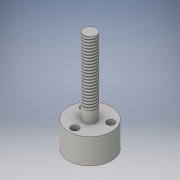
# Autodesk Inventor part: Motor top
Saved by Autodesk Inventor 2016 (Build 200138000, 138)
## iProperties
Created: 2015-05-11
Part Number: Motor top
Material: Generic
Document SubType Name: Modeling
Designer: Admin
Density: 1 g/cm^3
Appearance: Default
Author: Admin
Autodesk Inventor part; units mm, degrees
ref_plane "YZ Plane" through (0, 0, 0) normal (1, 0, 0) x (0, 1, 0)
ref_plane "XZ Plane" through (0, 0, 0) normal (0, 1, 0) x (-1, 0, 0)
ref_plane "XY Plane" through (0, 0, 0) normal (0, 0, 1) x (1, 0, 0)
sketch "Sketch1" plane through (0, 0, 0) normal (0, 1, 0) x (-1, 0, 0)
  circle A0 centre (0, 0) radius 8.5
  circle A1 centre (5.1962, -3) radius 1.5
  circle A2 centre (5.1962, -3) radius 1.5
  circle A3 centre (-5.1962, -3) radius 1.5
  circle A4 centre (-5.1962, -3) radius 1.5
  circle A5 centre (0, 6) radius 1.5
  circle A6 centre (0, 6) radius 1.5
  point P0 (0, 0)
  constraints: 7 centre point, 4 coincident
extrude "Extrusion1" add sketch "Sketch1" along normal blind 10
sketch "Sketch2" plane through (0, 10, 0) normal (0, 1, 0) x (1, 0, 0)
  circle A0 centre (0, 0) radius 2.5
  dimension "d3" = 5
  constraints: 1 centre point, 1 coincident
  measures "d3" diameter of A0
extrude "Extrusion2" add sketch "Sketch2" along normal blind 30
thread "Thread1" size "12-24 UNC" class "2A" standard "ANSI Unified Screw Threads" length 25.4
body "Solid1"
